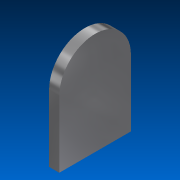
# Autodesk Inventor part: Terminal 2
Saved by Autodesk Inventor 2013 (Build 170138000, 138)
## iProperties
Created: 2012-05-07
Material: Copper
Document SubType Name: Modeling
Designer: sdarley
Density: 1 g/cm^3
Project: 2.1mm DC Power Socket
Description: Terminal 2
Author: sdarley
Title: Terminal 2
Revision Number: 1
Autodesk Inventor part; units mm, degrees
ref_plane "YZ Plane" through (0, 0, 0) normal (1, 0, 0) x (0, 1, 0)
ref_plane "XZ Plane" through (0, 0, 0) normal (0, 1, 0) x (-1, 0, 0)
ref_plane "XY Plane" through (0, 0, 0) normal (0, 0, 1) x (1, 0, 0)
sketch "Sketch1" plane through (0, 0, 0) normal (0, 0, 1) x (1, 0, 0)
  line L0 (-0.2, -1.4) -> (0.2, -1.4)
  line L1 (0.2, -1.4) -> (0.2, 1.4)
  line L2 (0.2, 1.4) -> (-0.2, 1.4)
  line L3 (-0.2, 1.4) -> (-0.2, -1.4)
  line L4 (-0.2, -1.4) -> (0.2, 1.4) construction
  line L5 (0.2, -1.4) -> (-0.2, 1.4) construction
  point P0 (0, 0)
  dimension "d0" = 0.4
  dimension "d1" = 2.8
  constraints: 12 end point, 2 midpoint, 2 parallel, 1 horizontal, 1 perpendicular
  measures "d0" distance of L2.end L1.end
  measures "d1" distance of L1.end L0.end
extrude "Extrusion1" add sketch "Sketch1" along normal blind 4
fillet "Fillet1" radius 1.4 2 edges at (0, -1.4, 4) (0, 1.4, 4)
body "Solid1"
